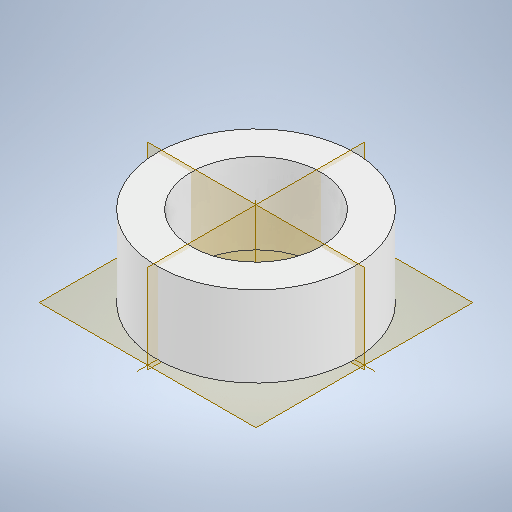
# Autodesk Inventor part: distance-ring
Saved by Autodesk Inventor 2025.2 (Build 292293000, 293)
## iProperties
Created: 2024-12-20
Part Number: distance-ring
Material: PC/ABS Plastic
Document SubType Name: Modeling
Designer: yehorderehus
Density: 1.1 g/cm^3
Appearance: Smooth - White
Mass: 0.293186 g
Surface Area: 3.87107 cm^2
Volume: 0.266533 cm^3
Author: yehorderehus
Autodesk Inventor part; units mm, degrees
sketch "Sketch1" plane through (0, 0, 0) normal (0, 1, 0) x (-1, 0, 0)
  circle A0 centre (0, 0) radius 6.1
  circle A1 centre (0, 0) radius 4
  dimension "d0" = 12.2
  dimension "d1" = 8
  constraints: 2 centre point, 2 coincident
  measures "d0" diameter of A0
  measures "d1" diameter of A1
extrude "Extrusion1" add sketch "Sketch1" along normal blind 5
body "Solid1"
